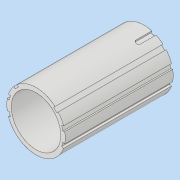
# Autodesk Inventor part: pistonTank
Saved by Autodesk Inventor 2017.3 (Build 213256000, 256)
## iProperties
Created: 2016-11-20
Part Number: pistonTank
Material: UHMW, White
Document SubType Name: Modeling
Designer: techn
Density: 0.94 g/cm^3
Appearance: Smooth - White
Mass: 207.673 g
Surface Area: 792.921 cm^2
Volume: 220.929 cm^3
Author: techn
Autodesk Inventor part; units mm, degrees
ref_plane "YZ Plane" through (0, 0, 0) normal (1, 0, 0) x (0, 1, 0)
ref_plane "XZ Plane" through (0, 0, 0) normal (0, 1, 0) x (-1, 0, 0)
ref_plane "XY Plane" through (0, 0, 0) normal (0, 0, 1) x (1, 0, 0)
sketch "Sketch1" plane through (0, 0, 0) normal (0, 0, 1) x (1, 0, 0)
  circle A0 centre (0, 0) radius 41.275
  circle A1 centre (0, 0) radius 34.925
  dimension "d0" = 82.55
  dimension "d1" = 69.85
  constraints: 2 centre point, 2 coincident
  measures "d0" diameter of A0
  measures "d1" diameter of A1
extrude "Extrusion1" add sketch "Sketch1" along normal blind 152.4
sketch "Sketch3" plane through (0, 0, 152.4) normal (0, 0, 1) x (1, 0, 0)
  line L0 (0, 0) -> (40.767, 0) construction
  line L1 (39.3779, -10.5513) -> (0, 0)
  line L2 (39.3779, -10.5513) -> (37.0103, -9.9169)
  line L3 (37.0103, -9.9169) -> (37.8321, -6.8501)
  line L4 (37.8321, -6.8501) -> (43.9657, -8.4936)
  line L5 (43.9657, -8.4936) -> (42.3222, -14.6272)
  line L6 (42.3222, -14.6272) -> (36.1886, -12.9837)
  line L7 (36.1886, -12.9837) -> (37.0103, -9.9169)
  dimension "d17" = 40.767
  dimension "d20" = 2.4511
  dimension "d21" = 6.35
  dimension "d22" = 6.35
  dimension "d28" = 15
  constraints: 16 end point, 4 perpendicular, 2 point on line, 1 collinear, 1 horizontal
  measures "d17" distance of L1.start L0.start
  measures "d20" distance of L1.start L2.end
  measures "d21" distance between parallel lines of L4 L6
  measures "d22" distance of L3.end L4.end
  measures "d28" angle of L1 L0
extrude "Extrusion5" cut sketch "Sketch3" against normal through all
pattern_circular "Circular Pattern2" count 3 over 60 about axis through (0, 0, 0) along (0, 0, 1) of "Extrusion5"
pattern_circular "Circular Pattern3" count 2 over 150 about axis through (0, 0, 0) along (0, 0, 1) of "Extrusion5", "Circular Pattern2"
sketch "Sketch6" plane through (0, 0, 0) normal (0, 0, -1) x (-1, 0, 0)
  line L0 (-16.0145, 34.7164) -> (-10.0474, 36.8882)
  line L1 (-10.0474, 36.8882) -> (-12.4199, 43.4065)
  line L2 (-12.4199, 43.4065) -> (-18.387, 41.2347)
  line L3 (-18.387, 41.2347) -> (-16.0145, 34.7164)
  line L4 (0, 0) -> (-13.031, 35.8023) construction
  line L5 (0, 0) -> (38.1, 0) construction
  dimension "d42" = 38.1
  dimension "d43" = 110
  dimension "d44" = 6.35
  constraints: 12 end point, 4 perpendicular, 1 equal length, 1 horizontal, 1 midpoint
  measures "d42" distance of L4.end L4.start
  measures "d43" angle of L5 L4
  measures "d44" distance between parallel lines of L1 L3
extrude "Extrusion7" cut sketch "Sketch6" against normal blind 25.4
fillet "Fillet1" radius 3.175 2 edges at (10.5695, 38.3225, 25.4) (16.5365, 36.1507, 25.4)
body "Solid1"
